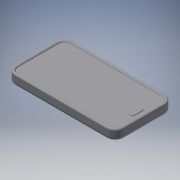
# Autodesk Inventor part: Samsung S5
Saved by Autodesk Inventor 2016 (Build 200138000, 138)
## iProperties
Created: 2016-11-04
Part Number: Samsung S5
Material: Generic
Document SubType Name: Modeling
Designer: william
Density: 1 g/cm^3
Appearance: Default
Author: william
Autodesk Inventor part; units mm, degrees
ref_plane "YZ Plane" through (0, 0, 0) normal (1, 0, 0) x (0, 1, 0)
ref_plane "XZ Plane" through (0, 0, 0) normal (0, 1, 0) x (-1, 0, 0)
ref_plane "XY Plane" through (0, 0, 0) normal (0, 0, 1) x (1, 0, 0)
sketch "Sketch1" plane through (0, 0, 0) normal (0, 0, 1) x (1, 0, 0)
  line L0 (12, 0) -> (134, 0)
  line L1 (146, 12) -> (146, 66)
  line L2 (134, 78) -> (12, 78)
  line L3 (0, 66) -> (0, 12)
  arc A0 (0, 12) -> (12, 0) centre (12, 12) ccw
  arc A1 (12, 78) -> (0, 66) centre (12, 66) ccw
  arc A2 (146, 66) -> (134, 78) centre (134, 66) ccw
  arc A3 (134, 0) -> (146, 12) centre (134, 12) ccw
  point P0 (0, 0)
  point P1 (146, 78)
  point P2 (146, 0)
  point P3 (0, 78)
  dimension "d0" = 78
  dimension "d1" = 146
  dimension "d5" = 12
  constraints: 8 end point, 8 point on circle, 8 point on line, 8 tangent, 4 centre point, 3 equal radius, 2 parallel, 1 horizontal, 1 perpendicular
  measures "d0" distance of point (146, 0) point (146, 78)
  measures "d1" distance of point (146, 78) point (0, 78)
  measures "d5" radius of A0
extrude "Extrusion1" add sketch "Sketch1" along normal blind 14
sketch "Sketch2" plane through (0, 0, 14) normal (0, 0, 1) x (1, 0, 0)
  line L0 (12, 0) -> (134, 0) projected
  line L1 (146, 12) -> (146, 66) projected
  line L2 (134, 78) -> (12, 78) projected
  line L3 (0, 66) -> (0, 12) projected
  arc A0 (0, 12) -> (12, 0) centre (12, 12) ccw projected
  arc A1 (134, 0) -> (146, 12) centre (134, 12) ccw projected
  arc A2 (146, 66) -> (134, 78) centre (134, 66) ccw projected
  arc A3 (12, 78) -> (0, 66) centre (12, 66) ccw projected
  line L4 (12, 74) -> (134, 74)
  arc A4 (142, 66) -> (134, 74) centre (134, 66) ccw
  line L5 (142, 66) -> (142, 12)
  arc A5 (134, 4) -> (142, 12) centre (134, 12) ccw
  line L6 (134, 4) -> (12, 4)
  arc A6 (4, 12) -> (12, 4) centre (12, 12) ccw
  line L7 (4, 12) -> (4, 66)
  arc A7 (12, 74) -> (4, 66) centre (12, 66) ccw
  point P0 (0, 0)
  dimension "d6" = 4
  constraints: 8 end point, 8 point on circle, 4 centre point, 7 other
  measures "d6" distance between parallel lines of L2 L4
extrude "Extrusion2" cut sketch "Sketch2" against normal blind 1.5 contours L4 A4 L5 A5 L6 A6 L7 A7
fillet "Fillet1" radius 2 16 edges at (139.6569, 71.6569, 14) (142, 39, 14) (139.6569, 6.3431, 14) (73, 4, 14) (6.3431, 6.3431, 14) (4, 39, 14) (6.3431, 71.6569, 14) (73, 74, 14) (3.5147, 74.4853, 14) (0, 39, 14) (3.5147, 3.5147, 14) (73, 0, 14) (142.4853, 3.5147, 14) (146, 39, 14) (142.4853, 74.4853, 14) (73, 78, 14)
sketch "Sketch3" plane through (0, 0, 0) normal (0, 0, -1) x (-1, 0, 0)
  line L0 (0, 12) -> (0, 66) projected
  arc A0 (0, 66) -> (-12, 78) centre (-12, 66) ccw projected
  line L1 (-12, 78) -> (-134, 78) projected
  arc A1 (-134, 78) -> (-146, 66) centre (-134, 66) ccw projected
  line L2 (-146, 66) -> (-146, 12) projected
  arc A2 (-146, 12) -> (-134, 0) centre (-134, 12) ccw projected
  line L3 (-134, 0) -> (-12, 0) projected
  arc A3 (-12, 0) -> (0, 12) centre (-12, 12) ccw projected
  circle A4 centre (-21, 39) radius 6.5
  line L4 (-13, 49.5) -> (-42, 49.5)
  line L5 (-44, 47.5) -> (-44, 30.5)
  line L6 (-42, 28.5) -> (-13, 28.5)
  line L7 (-11, 30.5) -> (-11, 47.5)
  arc A5 (-11, 47.5) -> (-13, 49.5) centre (-13, 47.5) ccw
  arc A6 (-42, 49.5) -> (-44, 47.5) centre (-42, 47.5) ccw
  arc A7 (-44, 30.5) -> (-42, 28.5) centre (-42, 30.5) ccw
  arc A8 (-13, 28.5) -> (-11, 30.5) centre (-13, 30.5) ccw
  point P0 (0, 0)
  point P1 (0, 39)
  point P2 (-11, 49.5)
  point P3 (-44, 28.5)
  point P4 (-11, 28.5)
  dimension "d10" = 13
  dimension "d11" = 21
  dimension "d12" = 33
  dimension "d13" = 21
  dimension "d14" = 10
  dimension "d15" = 10.5
  dimension "d16" = 2
  constraints: 8 end point, 8 point on circle, 8 tangent, 6 point on line, 5 centre point, 3 equal radius, 2 parallel, 1 horizontal, 1 horizontal alignment, 1 midpoint, 1 perpendicular
  measures "d10" diameter of A4
  measures "d11" distance from line of L0 A4.centre
  measures "d12" distance of point (-44, 28.5) point (-11, 28.5)
  measures "d13" distance of point (-11, 28.5) point (-11, 49.5)
  measures "d14" distance from line of A4.centre L7
  measures "d15" distance from line of L4 A4.centre
  measures "d16" radius of A5
extrude "Extrusion3" cut sketch "Sketch3" against normal blind 2 contours A5 L7 A8 L6 A7 L5 A6 L4
fillet "Fillet2" radius 2 9 edges at (27.5, 39, 0) (43.4142, 29.0858, 0) (44, 39, 0) (43.4142, 48.9142, 0) (27.5, 49.5, 0) (11.5858, 48.9142, 0) (11, 39, 0) (11.5858, 29.0858, 0) (27.5, 28.5, 0)
fillet "Fillet3" radius 4 8 edges at (142.4853, 74.4853, 0) (146, 39, 0) (142.4853, 3.5147, 0) (73, 0, 0) (3.5147, 3.5147, 0) (0, 39, 0) (3.5147, 74.4853, 0) (73, 78, 0)
sketch "Sketch4" plane through (0, 0, 12.5) normal (0, 0, 1) x (1, 0, 0)
  line L0 (134, 31) -> (136, 31)
  line L1 (138, 33) -> (138, 45)
  line L2 (136, 47) -> (134, 47)
  line L3 (132, 45) -> (132, 33)
  line L4 (142, 66) -> (142, 12) projected
  arc A0 (132, 33) -> (134, 31) centre (134, 33) ccw
  arc A1 (136, 31) -> (138, 33) centre (136, 33) ccw
  arc A2 (138, 45) -> (136, 47) centre (136, 45) ccw
  arc A3 (134, 47) -> (132, 45) centre (134, 45) ccw
  point P0 (0, 0)
  point P1 (132, 31)
  point P2 (138, 47)
  point P3 (132, 47)
  point P4 (138, 39)
  point P5 (142, 39)
  dimension "d21" = 16
  dimension "d22" = 6
  dimension "d23" = 4
  dimension "d24" = 2
  constraints: 8 end point, 8 point on circle, 8 tangent, 6 point on line, 4 centre point, 3 equal radius, 2 midpoint, 2 parallel, 1 horizontal, 1 horizontal alignment, 1 perpendicular
  measures "d21" distance of point (132, 47) point (132, 31)
  measures "d22" distance of point (138, 47) point (132, 47)
  measures "d23" distance between parallel lines of L4 L1
  measures "d24" radius of A0
extrude "Extrusion4" add sketch "Sketch4" along normal blind 1
fillet "Fillet4" radius 1 8 edges at (137.4142, 31.5858, 13.5) (138, 39, 13.5) (137.4142, 46.4142, 13.5) (135, 47, 13.5) (132.5858, 46.4142, 13.5) (132, 39, 13.5) (132.5858, 31.5858, 13.5) (135, 31, 13.5)
equation "\"d15\" = 0.5 * d13"
body "Solid1"
